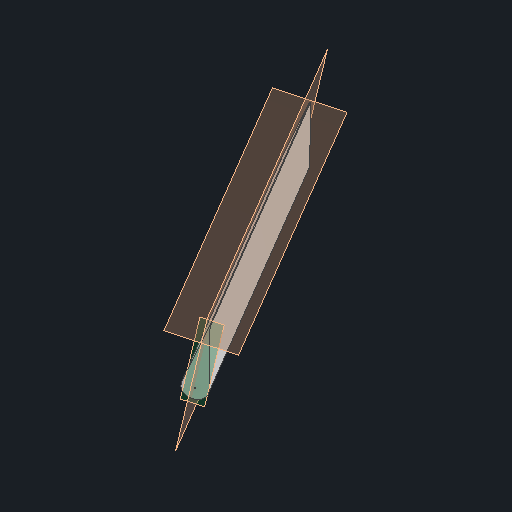
# Autodesk Inventor part: Vtail
Saved by Autodesk Inventor 2026.1 (Build 301233000, 233)
## iProperties
Created: 2025-08-11
Part Number: Vtail
Material: Generic
Document SubType Name: Modeling
Designer: Cupri
Density: 1 g/cm^3
Appearance: Default
Author: Cupri
Autodesk Inventor part; units mm, degrees
ref_plane "YZ Plane" through (0, 0, 0) normal (1, 0, 0) x (0, 1, 0)
ref_plane "XZ Plane" through (0, 0, 0) normal (0, 1, 0) x (-1, 0, 0)
ref_plane "Work Plane1" through (1169.1103, -81.3794, -3193.9196) normal (-0.4864, 0.0668, -0.8712) x (-0.8489, 0.1998, 0.4893)
sketch "Sketch1" plane through (1169.1103, -81.3794, -3193.9196) normal (-0.4864, 0.0668, -0.8712) x (-0.8489, 0.1998, 0.4893)
  circle A0 centre (-35.6307, -13.1161) radius 0.75 projected
  line L0 (-36.0087, 54.5034) -> (-35.2527, 54.5034) construction
  arc A1 (-48.6893, -20.4966) -> (-22.5721, -20.4966) centre (-35.6307, -13.1161) ccw construction
  arc A2 (-47.3555, -10.6379) -> (-23.9064, -10.636) centre (-35.6307, -13.1161) ccw
  line L1 (-47.5825, -12.2406) -> (-46.8097, -6.7847)
  line L2 (-23.6788, -12.2421) -> (-24.4519, -6.7847)
  line L3 (-47.5825, -12.2406) -> (-36.0087, 54.5034)
  line L4 (-36.0087, 54.5034) -> (-35.2527, 54.5034)
  line L5 (-35.2527, 54.5034) -> (-23.6788, -12.2421)
  spline S0 degree 3 poles (-35.2527, 54.5034) (-35.1874, 54.1932) (-35.0344, 53.4656) (-34.6342, 51.5408) (-34.4272, 50.5359) (-33.7132, 47.0386) (-33.2127, 44.5297) (-31.5162, 35.8392) (-30.3662, 29.6065) (-26.7707, 9.0774) (-24.4474, -5.9944) (-22.5721, -20.4966) knots -7.652768 -7.652768 -7.652768 -7.652768 -7.375677 -7.375677 -7.074889 -7.074889 -6.315253 -6.315253 -4.432937 -4.432937 -0.050389 -0.050389 -0.050389 -0.050389 projected
  spline S1 degree 3 poles (-48.6893, -20.4966) (-45.6503, 3.0044) (-41.2991, 29.0722) (-36.227, 53.4656) (-36.0741, 54.1932) (-36.0087, 54.5034) knots -2.513741 -2.513741 -2.513741 -2.513741 -0.095109 -0.095109 0 0 0 0 projected
  point P0 (2571.5058, -291.4034)
  constraints: 10 end point, 4 point on circle, 2 point on line, 1 centre point, 1 collinear
ref_plane "Work Plane2" through (-14.7431, -7.9324, 300) normal (0, 0, -1) x (0, 1, 0)
extrude "Extrusion1" add sketch "Sketch1" along normal blind 299.75 contours L3 L4 L5 A2
ref_plane "Work Plane4" through (1210.3037, -35.1412, -3213.3748) normal (0.8489, -0.1998, -0.4893) x (-0.4864, 0.0668, -0.8712)
ref_plane "Work Plane5" through (1210.6271, -35.2173, -3213.5612) normal (0.8489, -0.1998, -0.4893) x (-0.4864, 0.0668, -0.8712)
ref_plane "Work Plane6" through (1210.3037, -35.1412, -3213.3748) normal (0.2067, 0.9776, -0.0405) x (-0.4864, 0.0668, -0.8712)
body "Solid1"
